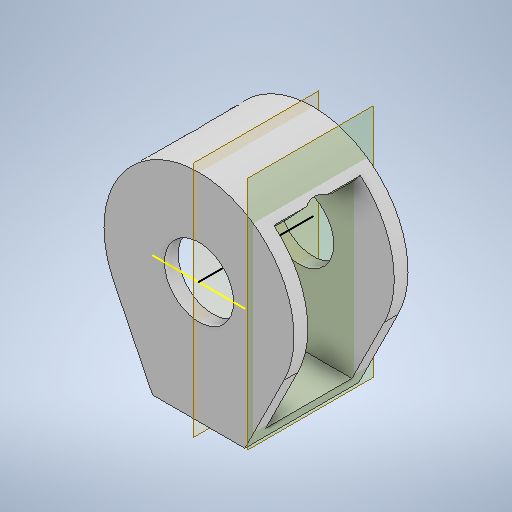
# Autodesk Inventor part: pulleyblocker
Saved by Autodesk Inventor 2025.2 (Build 292293000, 293)
## iProperties
Created: 2025-01-13
Part Number: pulleyblocker
Material: Generic
Document SubType Name: Modeling
Designer: email
Density: 1 g/cm^3
Appearance: Default
Author: email
Autodesk Inventor part; units mm, degrees
ref_plane "XZ Plane" through (0, 0, 0) normal (0, 1, 0) x (-1, 0, 0)
ref_plane "XY Plane" through (0, 0, 0) normal (0, 0, 1) x (1, 0, 0)
sketch "Sketch1" plane through (0, 0, 0) normal (0, 0, 1) x (1, 0, 0)
  line L0 (-13.5571, -30) -> (11.7429, -30) construction
  line L1 (11.7429, -30) -> (11.7429, -13.7014) construction
  line L2 (11.7429, -13.7014) -> (-13.5571, -13.7014) construction
  line L3 (-13.5571, -13.7014) -> (-13.5571, -30) construction
  circle A0 centre (0, 0) radius 10
  circle A1 centre (0, 0) radius 23.5 construction
  line L4 (11.7429, -30) -> (21.2173, -10.1032) construction
  line L5 (-13.5571, -30) -> (-21.9053, -8.5093) construction
  circle A2 centre (0, 0) radius 27.5
  line L6 (-13.4496, -35) -> (13.2752, -35)
  line L7 (-13.4496, -35) -> (-24.6844, -12.1216)
  line L8 (13.2752, -35) -> (24.6094, -12.273)
  dimension "d0" = 25.3
  dimension "d1" = 20
  dimension "d2" = 30
  dimension "d3" = 47
  dimension "d4" = 55
  dimension "d5" = 5
  constraints: 18 end point, 4 point on circle, 4 tangent, 3 centre point, 3 coincident, 2 horizontal, 2 parallel, 1 perpendicular
  measures "d0" distance between parallel lines of L1 L3
  measures "d1" diameter of A0
  measures "d2" distance from line of L0 A0.centre
  measures "d3" diameter of A1
  measures "d4" diameter of A2
  measures "d5" distance between parallel lines of L6 L0
extrude "Extrusion1" add sketch "Sketch1" along normal blind 4
sketch "Sketch2" plane through (0, 0, 4) normal (0, 0, 1) x (1, 0, 0)
  line L0 (-24.6844, -12.1216) -> (-13.4496, -35) projected
  line L1 (-13.4496, -35) -> (-15.4139, -31)
  line L2 (15.2701, -31) -> (-15.4139, -31)
  line L3 (13.2752, -35) -> (24.6094, -12.273) projected
  line L4 (15.2701, -31) -> (13.2752, -35)
  line L5 (-13.4496, -35) -> (13.2752, -35) projected
  line L6 (-13.4496, -35) -> (13.2752, -35)
  point P0 (0, 0)
  dimension "d8" = 4
  constraints: 8 end point, 2 collinear, 2 point on line, 1 horizontal
  measures "d8" distance between parallel lines of L5 L2
extrude "Extrusion2" add sketch "Sketch2" along normal blind 25
sketch "Sketch3" plane through (0, 0, 29) normal (0, 0, 1) x (1, 0, 0)
  line L0 (-13.5571, -30) -> (11.7429, -30) construction
  line L1 (11.7429, -30) -> (11.7429, -13.7014) construction
  line L2 (11.7429, -13.7014) -> (-13.5571, -13.7014) construction
  line L3 (-13.5571, -13.7014) -> (-13.5571, -30) construction
  circle A0 centre (0, 0) radius 10
  circle A1 centre (0, 0) radius 23.5 construction
  line L4 (11.7429, -30) -> (21.2173, -10.1032) construction
  line L5 (-13.5571, -30) -> (-21.9053, -8.5093) construction
  circle A2 centre (0, 0) radius 27.5
  line L6 (-13.4496, -35) -> (13.2752, -35)
  line L7 (-13.4496, -35) -> (-24.6844, -12.1216)
  line L8 (13.2752, -35) -> (24.6094, -12.273)
  dimension "d11" = 25.3
  dimension "d12" = 20
  dimension "d13" = 30
  dimension "d14" = 47
  dimension "d15" = 55
  dimension "d16" = 5
  constraints: 18 end point, 4 coincident, 4 point on circle, 4 tangent, 3 centre point, 2 horizontal, 2 parallel, 1 perpendicular
  measures "d11" distance between parallel lines of L1 L3
  measures "d12" diameter of A0
  measures "d13" distance from line of L0 A0.centre
  measures "d14" diameter of A1
  measures "d15" diameter of A2
  measures "d16" distance between parallel lines of L6 L0
extrude "Extrusion3" add sketch "Sketch3" along normal blind 4
sketch "Sketch4" plane through (0, 0, 0) normal (1, 0, 0) x (0, 1, 0)
  line L0 (-31, 4) -> (-31, 29) projected
  line L1 (16.3793, 67.7391) -> (20.3793, 67.7391) construction
  line L2 (20.3793, 44.4757) -> (20.3793, 67.7391) construction
  line L3 (20.3793, 44.4757) -> (16.3793, 44.4757) construction
  line L4 (0, 24) -> (0, 4)
  line L5 (16.3793, 44.4757) -> (16.3793, 48.4757) construction
  line L6 (16.3793, 67.7391) -> (16.3793, 63.7391) construction
  arc A0 (16.3793, 63.7391) -> (16.3793, 48.4757) centre (22.0199, 56.1074) ccw construction
  line L7 (27.5, 4) -> (-12.273, 4) projected
  line L8 (27.5, 4) -> (27.5, 29)
  line L9 (27.5, 29) -> (27.5, 33) projected
  line L10 (27.5, 29) -> (-12.273, 29) projected
  line L11 (27.5, 29) -> (24.5, 29)
  line L12 (24.5, 29) -> (24.5, 22.5)
  arc A1 (24.5, 22.5) -> (24.5, 10.5) centre (30.5208, 16.5) ccw
  line L13 (24.5, 10.5) -> (24.5, 4)
  line L14 (27.5, 4) -> (24.5, 4)
  point P0 (0, 0)
  point P1 (-12.1216, 29)
  point P2 (-12.1216, 4)
  point P3 (-12.273, 29)
  point P4 (24.5, 7.25)
  dimension "d22" = 4
  dimension "d23" = 4
  dimension "d24" = 4
  dimension "d25" = 3
  dimension "d26" = 6.5
  dimension "d27" = 3
  dimension "d28" = 6.5
  constraints: 22 end point, 4 point on circle, 3 vertical, 2 centre point, 2 collinear, 2 perpendicular, 2 point on line, 1 horizontal, 1 midpoint, 2 other
  measures "d22" distance of L3.end L5.end
  measures "d23" distance of L1.start L6.end
  measures "d24" distance between parallel lines of L2 L5
  measures "d25" distance between parallel lines of L12 L8
  measures "d26" distance of L11.end L12.end
  measures "d27" distance from line of L8 point (24.5, 7.25)
  measures "d28" distance of L13.start L13.end
revolve "Revolution1" add sketch "Sketch4" angle 80 mid plane about axis through (0, 0, 24) along (0, 0, -1)
sketch "Sketch5" plane through (0, 0, 0) normal (0, 1, 0) x (-1, 0, 0)
  line L0 (0, 0) -> (0.0872, 33)
  line L1 (13.4496, 33) -> (-13.2752, 33) projected
  constraints: 2 end point, 1 midpoint
sketch "Sketch7" plane through (0, 0, 0) normal (1, 0, 0) x (0, 1, 0)
  line L0 (28.8917, 11.9497) -> (28.8917, 21.0264) construction
  ellipse E0 centre (23.3803, 16.5) end of major axis (23.3803, 8) minor radius 6.5114 (18.7681, 22.5) -> (18.7681, 10.5) ccw projected
  line L1 (28.8917, 16.488) -> (29.8917, 16.488)
  arc A0 (28.8917, 11.9497) -> (28.8917, 21.0264) centre (45.4495, 16.488) ccw
  arc A1 (29.8597, 15.6582) -> (29.8917, 16.488) centre (23.0618, 16.3359) ccw
  line L2 (28.8917, 21.0264) -> (27.2308, 21.0264)
  line L3 (27.2308, 21.0264) -> (27.2308, 13.9093)
  line L4 (27.2308, 13.9093) -> (28.8917, 13.9093)
  line L5 (28.8917, 13.9093) -> (28.8917, 21.0264)
  point P0 (0, 0)
  point P1 (13.8599, 14.7128)
  point P2 (13.8237, 14.0101)
  point P3 (14.8237, 10.4516)
  dimension "d29" = 1
  constraints: 12 end point, 4 point on circle, 2 centre point, 2 horizontal, 2 parallel, 1 midpoint, 1 perpendicular, 1 vertical, 4 other
  measures "d29" distance of L1.end L1.start
extrude "Extrusion4" [suppressed]
sketch "Sketch9" plane through (-13.4496, -35, 0) normal (0, -1, 0) x (1, 0, 0)
  circle A0 centre (13.3624, 16.5) radius 5
  line L0 (0, 33) -> (26.7249, 33) projected
  line L1 (0, 0) -> (0, 33) projected
  line L2 (26.7249, 0) -> (26.7249, 33) projected
  line L3 (0, 0) -> (26.7249, 0) projected
  point P0 (13.4496, 0)
  dimension "d34" = 16.5
  dimension "d35" = 13.3624
  dimension "d36" = 26.7249
  dimension "d37" = 10
  dimension "d44" = 33
  constraints: 1 centre point
  measures "d34" distance from line of L0 A0.centre
  measures "d35" distance from line of L1 A0.centre
  measures "d36" distance between parallel lines of L1 L2
  measures "d37" diameter of A0
  measures "d44" distance between parallel lines of L3 L0
extrude "Extrusion5" cut sketch "Sketch9" against normal up to surface (4 mm away) contours A0
ref_plane "Work Plane1" through (15.7483, 18.7681, 29) normal (-1, 0, 0) x (0, 0, -1)
sketch "Sketch10" plane through (15.7483, 18.7681, 29) normal (-1, 0, 0) x (0, 0, -1)
  ellipse E0 centre (12.5, -4.6122) end of major axis (21, -4.6122) minor radius 6.5114 (18.5, 0) -> (6.5, 0) ccw projected
  line L0 (18.5, 0) -> (25, 0) projected
  arc A0 (6.5, 0) -> (18.5, 0) centre (12.5, 4.6778) ccw
  line L1 (0, 0) -> (0, -2.2981) projected
  line L2 (0, 0) -> (6.5, 0) projected
  ellipse E1 centre (12.5, -4.6122) end of major axis (21, -4.6122) minor radius 6.5114 (18.5, 0) -> (6.5, 0) ccw projected
  line L3 (18.5, 0) -> (25, 0) projected
  line L4 (25, -2.2981) -> (25, 0) projected
  line L5 (25, -2.2981) -> (0, -2.2981) projected
  arc A1 (18.5, 0) -> (6.5, 0) centre (12.5, -8.5282) ccw
  point P0 (29, 18.7681)
  point P1 (12.5, 1.8992)
  constraints: 4 point on circle, 2 centre point, 3 other
extrude "Extrusion6" cut sketch "Sketch10" along normal through all both and the other way through all contours A1 E0 | A0 L5 A1 | A1 E0 | A0 L5
mirror "Mirror1" about plane through (0, 0, 0) normal (1, 0, 0) of "Extrusion6"
equation "\"d35\" = 0.5 * d36"
body "Solid1"
